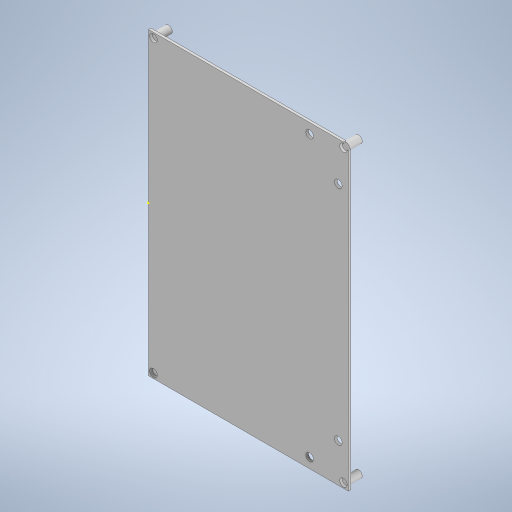
# Autodesk Inventor part: макетная плата
Saved by Autodesk Inventor 2023 (Build 270158000, 158)
## iProperties
Created: 2025-12-14
Part Number: макетная плата
Material: Типовые
Document SubType Name: Modeling
Designer: garin
Density: 1 g/cm^3
Appearance: По умолчанию
Author: garin
Autodesk Inventor part; units mm, degrees
ref_plane "YZ Plane" through (0, 0, 0) normal (1, 0, 0) x (0, 1, 0)
ref_plane "XZ Plane" through (0, 0, 0) normal (0, 1, 0) x (-1, 0, 0)
ref_plane "XY Plane" through (0, 0, 0) normal (0, 0, 1) x (1, 0, 0)
sketch "Эскиз2" plane through (0, 0, 0) normal (0, 0, 1) x (1, 0, 0)
  line L0 (80, 60) -> (0, 60)
  line L1 (0, 60) -> (0, -60)
  line L2 (0, -60) -> (80, -60)
  line L3 (80, -60) -> (80, 60)
  line L4 (80, 60) -> (78, 60)
  line L5 (78, 60) -> (78, 58)
  line L6 (78, 58) -> (80, 58)
  line L7 (80, 58) -> (80, 60)
  circle A0 centre (78, 58) radius 1.5
  line L8 (80, 0) -> (0, 0) construction
  circle A1 centre (78, -58) radius 1.5
  line L9 (40, 0) -> (40, 60) construction
  circle A2 centre (2, 58) radius 1.5
  circle A3 centre (2, -58) radius 1.5
  point P0 (79.5, 58)
  point P1 (78, 59.5)
  dimension "d5" = 120
  dimension "d6" = 2
  dimension "d7" = 2
  dimension "d8" = 3
  constraints: 20 end point, 4 centre point, 4 parallel, 4 symmetric about line, 3 horizontal, 3 midpoint, 2 coincident, 2 perpendicular, 3 other
  measures "d5" distance of L1.end L0.end
  measures "d6" distance of L6.end L5.end
  measures "d7" distance of L5.end L4.end
  measures "d8" diameter of A0
sketch "Эскиз3" plane through (0, 0, 0) normal (0, 0, 1) x (1, 0, 0)
  circle A0 centre (78, 57.9993) radius 1.5
  line L0 (79.5, 0) -> (0, 0)
  line L1 (0, 0) -> (40, 0) construction
  line L2 (40, 0) -> (40, 1.7902)
  line L3 (40, 1.7902) -> (40, 59.4993) construction
  circle A1 centre (78, -57.9993) radius 1.5
  circle A2 centre (2, 57.9993) radius 1.5
  circle A3 centre (2, -57.9993) radius 1.5
  dimension "d11" = 3
  dimension "d12" = 40
  constraints: 8 end point, 4 centre point, 3 symmetric about line, 2 point on line, 1 coincident, 1 horizontal, 3 other
  measures "d11" diameter of A0
  measures "d12" distance of L0.end L1.end
extrude "Выдавливание1" add sketch "Эскиз3" along normal blind 5
extrude "Выдавливание2" add sketch "Эскиз2" along normal blind 1 from surface at 5 contours L5 A0 L6 L3 L2 L1 L0
sketch "Эскиз4" plane through (0, -60, 6) normal (0, 0, 1) x (1, 0, 0)
  point P0 (0, 60)
sketch "Эскиз5" plane through (0, -60, 6) normal (0, 0, 1) x (1, 0, 0)
  circle A0 centre (78, 117.9993) radius 1.5 projected
  line L0 (78, 117.9993) -> (89, 117.9993) construction
  circle A1 centre (64.4943, 115.9487) radius 1.5
  circle A2 centre (75.9494, 104.4935) radius 1.5
  line L1 (80, 118) -> (80, 0) projected
  circle A3 centre (64.4943, 4.0513) radius 1.5
  circle A4 centre (75.9494, 15.5065) radius 1.5
  point P0 (0, 60)
  dimension "d21" = 3
  dimension "d22" = 3
  constraints: 4 centre point, 2 end point, 1 horizontal
  measures "d21" diameter of A1
  measures "d22" diameter of A2
extrude "Выдавливание3" cut sketch "Эскиз5" against normal blind 1 contours A1 | A2 | A3 | A4
